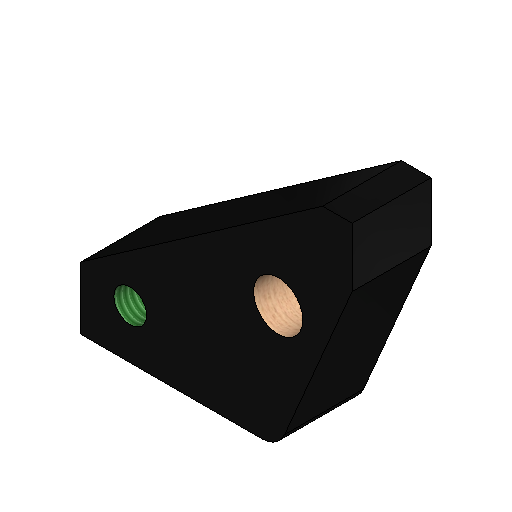
# Autodesk Inventor part: TL20240701-10100AT-003
Saved by Autodesk Inventor 2022.5 (Build 265521000, 521)
## iProperties
Category: ANTI BACK ASSY
Company: 현대트랜시스(대유)
RuleStatus: InUse
Part Number: TL20240701-10100AT-003
Project: SW-PJT
Checked By: 김형민
Engr Approved By: 김시현
User Status: 1 x78
Material: MC NYLON
Description: 0
Document SubType Name: Modeling
Mfg Approved By: 호상태
Designer: USER106
Stock Number: 003
Density: 0.94 g/cm^3
Appearance: Black
Detail Description: Processed products
Title: STOPPER BLOCK
Subject: SW차종 시트조립라인
Author: USER106
Revision Number: A
Autodesk Inventor part; units mm, degrees
ref_plane "YZ Plane" through (0, 0, 0) normal (1, 0, 0) x (0, 1, 0)
ref_plane "XZ Plane" through (0, 0, 0) normal (0, 1, 0) x (-1, 0, 0)
ref_plane "XY Plane" through (0, 0, 0) normal (0, 0, 1) x (1, 0, 0)
sketch "Sketch2" plane through (0, 0, 0) normal (0, 1, 0) x (-1, 0, 0)
  line L0 (-27.5, -23.5) -> (27.5, -23.5)
  line L1 (27.5, -23.5) -> (27.5, 23.5)
  line L2 (27.5, 23.5) -> (-27.5, 23.5)
  line L3 (-27.5, 23.5) -> (-27.5, -23.5)
  line L4 (-27.5, -23.5) -> (27.5, 23.5) construction
  line L5 (27.5, -23.5) -> (-27.5, 23.5) construction
  line L6 (27.5, -10.8102) -> (-21.5, 23.5)
  line L7 (-12.5, -23.5) -> (-27.5, 11.5)
  point P0 (0, 0)
  dimension "d1" = 55
  dimension "d2" = 47
  dimension "d3" = 15
  dimension "d4" = 6
  dimension "d5" = 35
  dimension "d28" = 35
  dimension "d29" = 12.6898
  constraints: 16 end point, 4 point on line, 2 midpoint, 2 parallel, 1 horizontal, 1 perpendicular
  measures "d1" distance of L2.end L1.end
  measures "d2" distance of L1.end L0.end
  measures "d3" horizontal distance of L7.start L7.end
  measures "d4" distance from line of L6.end L3
  measures "d5" vertical distance of L7.start L7.end
  measures "d28" angle of L2 L6
  measures "d29" distance from line of L6.start L0
extrude "Extrusion1" add sketch "Sketch2" along normal mid plane 16 contours L7 L3 L2 L6 L1 L0
sketch "Sketch3" plane through (0, -8, 0) normal (0, -1, 0) x (1, 0, 0)
  line L0 (-27.5, -23.5) -> (12.5, -23.5) projected
  line L1 (27.5, 11.5) -> (27.5, 23.5) projected
  point P0 (0, 0)
  point P1 (12.5, 1.5)
  dimension "d9" = 25
  dimension "d10" = 15
  measures "d9" distance from line of point (12.5, 1.5) L0
  measures "d10" distance from line of L1 point (12.5, 1.5)
hole "Hole1" at (12.5, -8, 1.5) direction (0, 1, 0) diameter 10 end through all
sketch "Sketch4" plane through (0, -8, 0) normal (0, -1, 0) x (1, 0, 0)
  line L0 (-27.5, -23.5) -> (12.5, -23.5) projected
  line L1 (27.5, 11.5) -> (27.5, 23.5) projected
  point P0 (0, 0)
  point P1 (-17.5, -13.5)
  dimension "d18" = 10
  dimension "d19" = 45
  measures "d18" distance from line of point (-17.5, -13.5) L0
  measures "d19" distance from line of L1 point (-17.5, -13.5)
hole "Hole2" at (-17.5, -8, -13.5) direction (0, 1, 0) diameter 6.647 end through all thread size "M8x1.25" class "6H" standard "TS profile"
fillet "Fillet1" radius 5 1 edges at (12.5, 0, -23.5)
body "Solid1"
